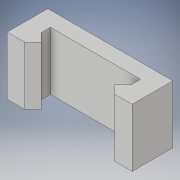
# Autodesk Inventor part: clip3
Saved by Autodesk Inventor 2019.3 (Build 233278000, 278)
## iProperties
Created: 2019-04-12
Part Number: clip3
Material: Generic
Document SubType Name: Modeling
Designer: peter
Density: 1 g/cm^3
Appearance: Default
Author: peter
Autodesk Inventor part; units mm, degrees
ref_plane "YZ Plane" through (0, 0, 0) normal (1, 0, 0) x (0, 1, 0)
ref_plane "XZ Plane" through (0, 0, 0) normal (0, 1, 0) x (-1, 0, 0)
ref_plane "XY Plane" through (0, 0, 0) normal (0, 0, 1) x (1, 0, 0)
sketch "Sketch1" plane through (0, 0, 0) normal (0, 1, 0) x (-1, 0, 0)
  line L0 (0, 0) -> (15.5, 0)
  line L1 (0, 0) -> (0, 1.6)
  line L2 (0, 1.6) -> (1.4142, 3.0142)
  line L3 (1.4142, 3.0142) -> (0, 4.4284)
  line L4 (0, 4.4284) -> (-3, 4.4284)
  line L5 (-3, 4.4284) -> (-3, -2.5716)
  line L6 (0, 0) -> (7.5, 0) construction
  line L7 (7.5, 0) -> (7.5, 8.2987) construction
  line L8 (15.5, 0) -> (15.5, 1.6)
  line L9 (15.5, 1.6) -> (14.0858, 3.0142)
  line L10 (14.0858, 3.0142) -> (15.5, 4.4284)
  line L11 (15.5, 4.4284) -> (18.5, 4.4284)
  line L12 (18.5, 4.4284) -> (18.5, -2.5716)
  line L13 (18.5, -2.5716) -> (-3, -2.5716)
  dimension "d0" = 15.5
  dimension "d1" = 1.6
  dimension "d2" = 2
  dimension "d3" = 135
  dimension "d4" = 2
  dimension "d5" = 3
  dimension "d6" = 7
  dimension "d7" = 7.5
  dimension "d8" = 1.6
  dimension "d9" = 2
  dimension "d10" = 135
  dimension "d11" = 2
  dimension "d12" = 3
  dimension "d13" = 7
  constraints: 28 end point, 4 perpendicular, 3 point on line, 3 vertical, 1 horizontal
  measures "d0" distance of L0.start L0.end
  measures "d1" distance of L0.start L1.end
  measures "d2" distance of L1.end L2.end
  measures "d3" angle of L1 L2
  measures "d4" distance of L2.end L3.end
  measures "d5" distance of L3.end L4.end
  measures "d6" distance of L4.end L5.end
  measures "d7" distance of L0.start L6.end
  measures "d8" distance of L0.end L8.end
  measures "d9" distance of L8.end L9.end
  measures "d10" angle of L9 L8
  measures "d11" distance of L9.end L10.end
  measures "d12" distance of L10.end L11.end
  measures "d13" distance of L11.end L12.end
extrude "Extrusion1" add sketch "Sketch1" along normal blind 10
body "Solid1"
